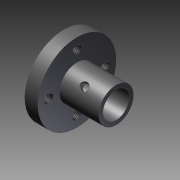
# Autodesk Inventor part: SSTHRT12-MB_b
Saved by Autodesk Inventor 2011 SP1 (Build 150282100, 282)
## iProperties
Created: 2016-04-10
Part Number: SSTHRT12-MB_b
Catalog Web Link: www.cadenas.de
Description: STHRBT, STHRT,  SSTHRT_b-Shaft Supports - Bracket Shaped - Standard Tapped Mounting Hole Type - Round Flange
Vendor: MISUMI
Document SubType Name: Modeling
Designer: psAdmin
Manufacturer: MISUMI
Mass: 6.7735 g
Surface Area: 44.6396 cm^2
Volume: 6.7735 cm^3
Density: 1 g/cm^3
Category: PARTsolutions
Company: MISUMI
Title: SSTHRT12-MB
Author: Cadenas PARTsolutions
Comments: Shaft Supports - Bracket Shaped - Standard Tapped Mounting Hole Type - Round Flange
PSOL_IDENT_0: {$CADENAS_DATA\23d-libs\misumi\metric\02_shaft_supports\ssthrt\ssthrt_body.prj},194 {VTYP=3D},{NB=SS
PSOL_IDENT_1: THRT12-MB_b},{LINA=SSTHRT12-MB},{NN=STHRBT, STHRT,  SSTHRT_b},{DATE=21.05.2015 00:56:56},{GEOMDATE=2
PSOL_IDENT_2: 1.05.2015 00:56:56},{VERSION=},{LINEID=70},{LINESUBID=-1},{WBVAR=MAT,ST,ALT}  {NB=SSTHRT12-MB_b},{LI
PSOL_IDENT_3: NA=SSTHRT12-MB},{KT=DUMMY},{PN=SSTHRT12-MB},{TS=2},{TSALG= '1', 'Drilled Mounting Hole', '2', 'Tappe
PSOL_IDENT_4: d Mounting Hole' },{TYPE=SSTHRT},{MAT=304},{MATA= '1018', 'SS400 Equivalent', '304', 'SUS304' },{MAL
PSOL_IDENT_5: G='M4'},{ST=-},{ST0= '-','-' },{D=12},{THMD11='M4'},{THMD13='M4'},{THMD12='M4'},{DTOL=+0.018/0},{DX=
PSOL_IDENT_6: 12},{N=2.0},{L=24},{D1=16},{H=36},{T=6.0},{LL=15},{M=M4},{THMD=4},{THMD1=M4},{THMD2=M4},{P=26},{K=28
PSOL_IDENT_7: },{W=20},{P1=26},{F=0},{DD1=4.5},{DD11=4.5},{DD12=4.5},{M1=M4},{M11=4},{ALT=MB},{ALTPN=-MB},{BM=4},{
PSOL_IDENT_8: BL=3}
NN: STHRBT, STHRT,  SSTHRT_b
NT: Shaft Supports - Bracket Shaped - Standard Tapped Mounting Hole Type - Round Flange
NB: SSTHRT12-MB_b
NBSYN: $PN._b
LINA: SSTHRT12-MB
PN: SSTHRT12-MB
MAT: SUS304
ST: -
D: 12
DTOL: +0.018/0
N: 2.0
L: 24
D1: 16
H: 36
T: 6.0
LL: 15
M: M4
P: 26
M1: M4
ALT: with MB (Hex Socket Set Screw Included)
SUPPLIER: MISUMI
ARTICLENO: SSTHRT12-MB_b
BOMINFO: SSTHRT12-MB
CREATOR: CADENAS GmbH
Autodesk Inventor part; units mm, degrees
sketch "Sketch_1" plane through (0, 0, 0) normal (0, 0, 1) x (1, 0, 0)
  line L0 (24, 0) -> (0, 0)
  line L1 (0, 18) -> (0, 6)
  line L2 (0, 6) -> (24, 6)
  line L3 (24, 6) -> (24, 8)
  line L4 (24, 8) -> (6, 8)
  line L5 (6, 8) -> (6, 18)
  line L6 (6, 18) -> (0, 18)
  constraints: 14 end point
revolve "Revolution1" add sketch "Sketch_1" angle 360 about axis through (24, 0, 0) along (1, 0, 0)
sketch "Sketch_3" plane through (0, 0, 0) normal (0, -0.7071, 0.7071) x (1, 0, 0)
  line L0 (15, 5.5) -> (15, 8)
  line L1 (15, 8) -> (17, 8)
  line L2 (17, 8) -> (16.621, 7.621)
  line L3 (16.621, 7.621) -> (16.621, 5.5)
  line L4 (16.621, 5.5) -> (15, 5.5)
  line L5 (15, 5.5) -> (15, 8)
  constraints: 12 end point
revolve "Revolution2" cut sketch "Sketch_3" angle 360 about axis through (15, 3.8891, 3.8891) along (0, -0.7071, -0.7071)
thread "Thread1" size "M4x0.7" class "6H" standard "ISO Metric profile" length 2.121
sketch "Sketch_2" plane through (0, 0, 0) normal (0, -0.7071, -0.7071) x (1, 0, 0)
  line L0 (15, 5.5) -> (15, 8)
  line L1 (15, 8) -> (17, 8)
  line L2 (17, 8) -> (16.621, 7.621)
  line L3 (16.621, 7.621) -> (16.621, 5.5)
  line L4 (16.621, 5.5) -> (15, 5.5)
  line L5 (15, 5.5) -> (15, 8)
  constraints: 12 end point
revolve "Revolution3" cut sketch "Sketch_2" angle 360 about axis through (15, -3.8891, 3.8891) along (0, 0.7071, -0.7071)
thread "Thread2" size "M4x0.7" class "6H" standard "ISO Metric profile" length 2.121
sketch "Sketch_4" plane through (0, 0, 0) normal (0, 0, 1) x (1, 0, 0)
  line L0 (6, 13) -> (0, 13)
  line L1 (0, 13) -> (0, 15)
  line L2 (0, 15) -> (0.379, 14.621)
  line L3 (0.379, 14.621) -> (5.621, 14.621)
  line L4 (5.621, 14.621) -> (6, 15)
  line L5 (6, 15) -> (6, 13)
  line L6 (6, 13) -> (0, 13)
  constraints: 14 end point
revolve "Revolution4" cut sketch "Sketch_4" angle 360 about axis through (6, 13, 0) along (1, 0, 0)
thread "Thread3" size "M4x0.7" class "6H" standard "ISO Metric profile" full length
sketch "Sketch_9" plane through (0, 0, 0) normal (0, -1, 0) x (1, 0, 0)
  line L0 (0, -13) -> (6, -13)
  line L1 (6, -13) -> (6, -15)
  line L2 (6, -15) -> (5.621, -14.621)
  line L3 (5.621, -14.621) -> (0.379, -14.621)
  line L4 (0.379, -14.621) -> (0, -15)
  line L5 (0, -15) -> (0, -13)
  line L6 (0, -13) -> (6, -13)
  constraints: 14 end point
revolve "Revolution5" cut sketch "Sketch_9" angle 360 about axis through (0, 0, -13) along (-1, 0, 0)
thread "Thread4" size "M4x0.7" class "6H" standard "ISO Metric profile" full length
sketch "Sketch_10" plane through (0, 0, 0) normal (0, 0, 1) x (1, 0, 0)
  line L0 (0, -13) -> (6, -13)
  line L1 (6, -13) -> (6, -15)
  line L2 (6, -15) -> (5.621, -14.621)
  line L3 (5.621, -14.621) -> (0.379, -14.621)
  line L4 (0.379, -14.621) -> (0, -15)
  line L5 (0, -15) -> (0, -13)
  line L6 (0, -13) -> (6, -13)
  constraints: 14 end point
revolve "Revolution6" cut sketch "Sketch_10" angle 360 about axis through (0, -13, 0) along (-1, 0, 0)
thread "Thread5" size "M4x0.7" class "6H" standard "ISO Metric profile" full length
sketch "Sketch_11" plane through (0, 0, 0) normal (0, -1, 0) x (1, 0, 0)
  line L0 (6, 13) -> (0, 13)
  line L1 (0, 13) -> (0, 15)
  line L2 (0, 15) -> (0.379, 14.621)
  line L3 (0.379, 14.621) -> (5.621, 14.621)
  line L4 (5.621, 14.621) -> (6, 15)
  line L5 (6, 15) -> (6, 13)
  line L6 (6, 13) -> (0, 13)
  constraints: 14 end point
revolve "Revolution7" cut sketch "Sketch_11" angle 360 about axis through (6, 0, 13) along (1, 0, 0)
thread "Thread6" size "M4x0.7" class "6H" standard "ISO Metric profile" full length
ref_plane "to_screw1_XY" through (15, 4.2426, 4.2426) normal (0, 0.7071, 0.7071) x (1, 0, 0)
ref_plane "to_screw1_YZ" through (15, 4.2426, 4.2426) normal (1, 0, 0) x (0, 0.7071, -0.7071)
ref_plane "to_screw1_ZX" through (15, 4.2426, 4.2426) normal (0, 0.7071, -0.7071) x (0, 0.7071, 0.7071)
ref_plane "to_screw2_XY" through (15, -4.2426, 4.2426) normal (0, -0.7071, 0.7071) x (1, 0, 0)
ref_plane "to_screw2_YZ" through (15, -4.2426, 4.2426) normal (1, 0, 0) x (0, 0.7071, 0.7071)
ref_plane "to_screw2_ZX" through (15, -4.2426, 4.2426) normal (0, 0.7071, 0.7071) x (0, -0.7071, 0.7071)
body "Solid1"
